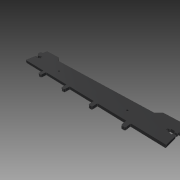
# Autodesk Inventor part: frame_brace_top
Saved by Autodesk Inventor 2014 (Build 180170000, 170)
## iProperties
Created: 2013-12-06
Part Number: frame_brace_top
Material: Plywood, Finish
Document SubType Name: Modeling
Designer: buben
Density: 0.552 g/cm^3
Appearance: Plywood - New
Author: buben
Subject: Laser Cutted
Autodesk Inventor part; units mm, degrees
ref_plane "YZ Plane" through (0, 0, 0) normal (1, 0, 0) x (0, 1, 0)
ref_plane "XZ Plane" through (0, 0, 0) normal (0, 1, 0) x (-1, 0, 0)
ref_plane "XY Plane" through (0, 0, 0) normal (0, 0, 1) x (1, 0, 0)
sketch "Sketch1" plane through (0, 0, 0) normal (0, 0, 1) x (1, 0, 0)
  line L0 (0, 0) -> (336, 0)
  line L1 (336, 0) -> (336, 55)
  line L2 (0, 55) -> (0, 0)
  line L3 (40, 55) -> (50, 45)
  line L4 (50, 45) -> (286, 45)
  line L5 (286, 45) -> (296, 55)
  line L6 (336, 55) -> (296, 55)
  line L7 (40, 55) -> (0, 55)
  dimension "d0" = 336
  dimension "d1" = 55
  dimension "d2" = 45
  dimension "d3" = 40
  dimension "d4" = 10
  dimension "d5" = 40
  constraints: 16 end point, 3 parallel, 3 perpendicular, 1 collinear, 1 horizontal
  measures "d0" distance of L0.start L0.end
  measures "d1" distance of L2.start L0.start
  measures "d2" angle of L7 L3
  measures "d3" distance of L3.start L2.start
  measures "d4" distance between parallel lines of L7 L4
  measures "d5" distance of L1.end L5.end
extrude "Extrusion1" add sketch "Sketch1" along normal blind 6.5
sketch "Sketch2" plane through (0, 0, 6.5) normal (0, 0, 1) x (1, 0, 0)
  line L0 (0, 0) -> (336, 0) projected
  line L1 (286, 45) -> (50, 45) projected
  line L2 (0, 55) -> (0, 0) projected
  line L3 (0, 25.25) -> (0, 29.75)
  line L4 (16.3, 29.75) -> (16.3, 25.25)
  line L5 (5, 32.25) -> (12.3, 32.25)
  line L6 (12.3, 22.75) -> (5, 22.75)
  line L7 (0, 29.75) -> (5, 29.75)
  line L8 (12.3, 29.75) -> (16.3, 29.75)
  line L9 (16.3, 25.25) -> (12.3, 25.25)
  line L10 (5, 25.25) -> (0, 25.25)
  line L11 (5, 22.75) -> (5, 25.25)
  line L12 (5, 29.75) -> (5, 32.25)
  line L13 (12.3, 32.25) -> (12.3, 29.75)
  line L14 (12.3, 25.25) -> (12.3, 22.75)
  line L15 (168, 0) -> (168, 45) construction
  line L16 (336, 25.25) -> (336, 29.75)
  line L17 (319.7, 29.75) -> (319.7, 25.25)
  line L18 (331, 32.25) -> (323.7, 32.25)
  line L19 (323.7, 22.75) -> (331, 22.75)
  line L20 (336, 29.75) -> (331, 29.75)
  line L21 (323.7, 29.75) -> (319.7, 29.75)
  line L22 (319.7, 25.25) -> (323.7, 25.25)
  line L23 (331, 25.25) -> (336, 25.25)
  line L24 (331, 22.75) -> (331, 25.25)
  line L25 (331, 29.75) -> (331, 32.25)
  line L26 (323.7, 32.25) -> (323.7, 29.75)
  line L27 (323.7, 25.25) -> (323.7, 22.75)
  point P0 (0, 27.5)
  point P1 (0, 27.5)
  point P2 (336, 27.5)
  point P3 (336, 27.5)
  dimension "d8" = 4.5
  dimension "d9" = 2.5
  dimension "d10" = 2.5
  dimension "d11" = 5
  dimension "d12" = 7.3
  dimension "d13" = 4
  constraints: 50 end point, 14 symmetric about line, 10 parallel, 5 collinear, 4 midpoint, 4 perpendicular, 3 horizontal, 1 coincident
  measures "d8" distance of L4.start L4.end
  measures "d9" distance of L5.end L8.start
  measures "d10" distance of L9.end L6.start
  measures "d11" distance of L10.start L3.start
  measures "d12" distance of L6.start L6.end
  measures "d13" distance of L4.end L9.end
extrude "Extrusion2" cut sketch "Sketch2" against normal through all
sketch "Sketch3" plane through (0, 0, 6.5) normal (0, 0, 1) x (1, 0, 0)
  line L0 (0, 25.25) -> (0, 0) projected
  line L1 (0, 0) -> (336, 0) projected
  line L2 (336, 0) -> (336, 25.25) projected
  line L3 (336, 29.75) -> (336, 55) projected
  line L4 (0, 55) -> (0, 29.75) projected
  line L5 (16.3, 29.75) -> (16.3, 25.25) projected
  line L6 (0, 43) -> (-4.5, 43)
  line L7 (-6.5, 41) -> (-6.5, 37)
  line L8 (-4.5, 35) -> (0, 35)
  line L9 (0, 35) -> (0, 43)
  line L10 (0, 20) -> (-4.5, 20)
  line L11 (-6.5, 18) -> (-6.5, 14)
  line L12 (-4.5, 12) -> (0, 12)
  line L13 (0, 12) -> (0, 20)
  arc A0 (-4.5, 43) -> (-6.5, 41) centre (-4.5, 41) ccw
  arc A1 (-6.5, 37) -> (-4.5, 35) centre (-4.5, 37) ccw
  arc A2 (-4.5, 20) -> (-6.5, 18) centre (-4.5, 18) ccw
  arc A3 (-6.5, 14) -> (-4.5, 12) centre (-4.5, 14) ccw
  line L14 (336, 43) -> (340.5, 43)
  line L15 (342.5, 41) -> (342.5, 37)
  line L16 (340.5, 35) -> (336, 35)
  line L17 (336, 35) -> (336, 43)
  line L18 (336, 20) -> (340.5, 20)
  line L19 (342.5, 18) -> (342.5, 14)
  line L20 (340.5, 12) -> (336, 12)
  line L21 (336, 12) -> (336, 20)
  arc A4 (342.5, 41) -> (340.5, 43) centre (340.5, 41) ccw
  arc A5 (340.5, 35) -> (342.5, 37) centre (340.5, 37) ccw
  arc A6 (342.5, 18) -> (340.5, 20) centre (340.5, 18) ccw
  arc A7 (340.5, 12) -> (342.5, 14) centre (340.5, 14) ccw
  line L22 (198.4, 0) -> (206.4, 0)
  line L23 (206.4, 0) -> (206.4, -11)
  line L24 (204.4, -13) -> (200.4, -13)
  line L25 (198.4, -11) -> (198.4, 0)
  line L26 (137.6, 0) -> (129.6, 0)
  line L27 (129.6, 0) -> (129.6, -11)
  line L28 (131.6, -13) -> (135.6, -13)
  line L29 (137.6, -11) -> (137.6, 0)
  line L30 (60.8, 0) -> (68.8, 0)
  line L31 (68.8, 0) -> (68.8, -11)
  line L32 (66.8, -13) -> (62.8, -13)
  line L33 (60.8, -11) -> (60.8, 0)
  line L34 (267.2, 0) -> (275.2, 0)
  line L35 (275.2, 0) -> (275.2, -11)
  line L36 (273.2, -13) -> (269.2, -13)
  line L37 (267.2, -11) -> (267.2, 0)
  arc A8 (60.8, -11) -> (62.8, -13) centre (62.8, -11) ccw
  arc A9 (66.8, -13) -> (68.8, -11) centre (66.8, -11) ccw
  arc A10 (129.6, -11) -> (131.6, -13) centre (131.6, -11) ccw
  arc A11 (135.6, -13) -> (137.6, -11) centre (135.6, -11) ccw
  arc A12 (198.4, -11) -> (200.4, -13) centre (200.4, -11) ccw
  arc A13 (204.4, -13) -> (206.4, -11) centre (204.4, -11) ccw
  arc A14 (267.2, -11) -> (269.2, -13) centre (269.2, -11) ccw
  arc A15 (273.2, -13) -> (275.2, -11) centre (273.2, -11) ccw
  line L38 (68.8, -5.5) -> (129.6, -5.5) construction
  line L39 (137.6, -5.5) -> (198.4, -5.5) construction
  line L40 (206.4, -5.5) -> (267.2, -5.5) construction
  line L41 (275.2, -5.5) -> (336, -5.5) construction
  line L42 (60.8, -5.5) -> (0, -5.5) construction
  point P0 (16.3, 27.5)
  point P1 (168, 0)
  dimension "d16" = 2
  dimension "d17" = 8
  dimension "d18" = 8
  dimension "d19" = 15
  dimension "d20" = 7.5
  dimension "d21" = 6.5
  dimension "d22" = 2
  dimension "d23" = 6.5
  dimension "d24" = 2
  dimension "d25" = 8
  dimension "d26" = 8
  dimension "d27" = 8
  dimension "d28" = 8
  dimension "d29" = 13
  constraints: 74 end point, 32 point on circle, 32 tangent, 16 centre point, 16 parallel, 15 collinear, 13 equal radius, 10 midpoint, 8 horizontal, 8 perpendicular, 8 point on line, 2 vertical alignment
  measures "d16" radius of A0
  measures "d17" distance between parallel lines of L12 L10
  measures "d18" distance between parallel lines of L6 L8
  measures "d19" distance between parallel lines of L10 L8
  measures "d20" distance from line of point (16.3, 27.5) L8
  measures "d21" distance between parallel lines of L4 L7
  measures "d22" radius of A4
  measures "d23" distance between parallel lines of L3 L15
  measures "d24" radius of A8
  measures "d25" distance between parallel lines of L31 L33
  measures "d26" distance between parallel lines of L29 L27
  measures "d27" distance between parallel lines of L23 L25
  measures "d28" distance between parallel lines of L35 L37
  measures "d29" distance between parallel lines of L1 L32
extrude "Extrusion3" add sketch "Sketch3" against normal blind 6.5
sketch "Sketch4" plane through (0, 0, 6.5) normal (0, 0, 1) x (1, 0, 0)
  line L0 (0, 20) -> (-4.5, 20) projected
  arc A0 (-4.5, 20) -> (-6.5, 18) centre (-4.5, 18) ccw projected
  line L1 (-6.5, 18) -> (-6.5, 14) projected
  arc A1 (-6.5, 14) -> (-4.5, 12) centre (-4.5, 14) ccw projected
  line L2 (-4.5, 12) -> (0, 12) projected
  line L3 (336, 12) -> (340.5, 12) projected
  arc A2 (340.5, 12) -> (342.5, 14) centre (340.5, 14) ccw projected
  line L4 (342.5, 14) -> (342.5, 18) projected
  arc A3 (342.5, 18) -> (340.5, 20) centre (340.5, 18) ccw projected
  line L5 (340.5, 20) -> (336, 20) projected
  line L6 (5, 22.75) -> (5, 25.25) projected
  line L7 (0, 20) -> (0, 12)
  line L8 (336, 20) -> (336, 12)
  constraints: 4 end point, 2 parallel
extrude "Extrusion4" cut sketch "Sketch4" against normal through all
sketch "Sketch5" plane through (0, 0, 6.5) normal (0, 0, 1) x (1, 0, 0)
  line L0 (0, 25.25) -> (0, 0) projected
  line L1 (0, 0) -> (60.8, 0) projected
  line L2 (336, 0) -> (336, 25.25) projected
  circle A0 centre (83.25, 20) radius 2.25
  circle A1 centre (252.75, 20) radius 2.25
  dimension "d34" = 4.5
  dimension "d35" = 20
  dimension "d36" = 83.25
  dimension "d37" = 83.25
  constraints: 2 centre point, 1 equal radius, 1 horizontal alignment
  measures "d34" diameter of A0
  measures "d35" distance from line of L1 A0.centre
  measures "d36" distance from line of L0 A0.centre
  measures "d37" distance from line of L2 A1.centre
extrude "Extrusion5" cut sketch "Sketch5" against normal through all
equation "\"d5\" = d3"
equation "\"d23\" = d21"
equation "\"d37\" = d36"
body "Solid1"
